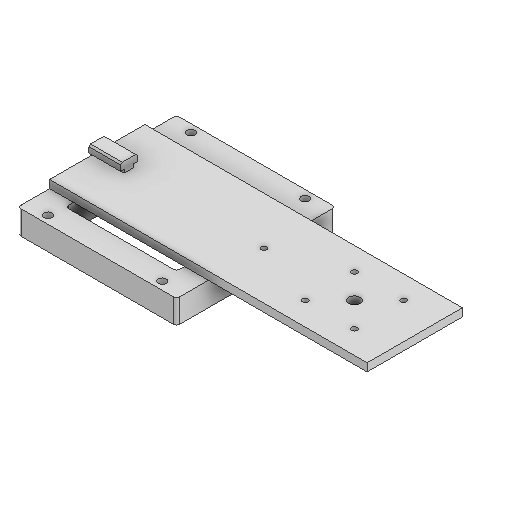
# Autodesk Inventor part: podstawka_prowadzaca
Saved by Autodesk Inventor 2025.1 (Build 291241000, 241)
## iProperties
Created: 2025-03-27
Part Number: podstawka_prowadzaca
Material: Ogólny
Document SubType Name: Modeling
Designer: Maciej
Density: 1 g/cm^3
Appearance: Domyślna
Author: Maciej
Autodesk Inventor part; units mm, degrees
ref_plane "YZ Plane" through (0, 0, 0) normal (1, 0, 0) x (0, 1, 0)
ref_plane "XZ Plane" through (0, 0, 0) normal (0, 1, 0) x (-1, 0, 0)
ref_plane "XY Plane" through (0, 0, 0) normal (0, 0, 1) x (1, 0, 0)
sketch "Szkic1" plane through (0, 0, 0) normal (0, 1, 0) x (-1, 0, 0)
  line L0 (0, 0) -> (100, 0)
  line L1 (100, 0) -> (100, -100)
  line L2 (100, -100) -> (0, -100)
  line L3 (0, -100) -> (0, 0)
  dimension "d0" = 100
  dimension "d1" = 100
  constraints: 8 end point, 2 parallel, 1 horizontal, 1 perpendicular
  measures "d0" distance of L0.end L1.end
  measures "d1" distance of L1.end L2.end
sketch "Szkic2" plane through (0, 0, 0) normal (0, 1, 0) x (-1, 0, 0)
  line L0 (15, -15) -> (85, -15)
  line L1 (85, -15) -> (85, -85)
  line L2 (85, -85) -> (15, -85)
  line L3 (15, -85) -> (15, -15)
  point P0 (0, 0)
  dimension "d2" = 70
  dimension "d3" = 70
  dimension "d4" = 15
  dimension "d5" = 15
  constraints: 8 end point, 2 parallel, 1 horizontal, 1 perpendicular
  measures "d2" distance of L1.end L2.end
  measures "d3" distance of L0.end L1.end
  measures "d4" horizontal distance of point (0, 0) L0.start
  measures "d5" horizontal distance of point (0, 0) L0.start
extrude "Wyciągnięcie proste1" add sketch "Szkic1" along normal blind 15
extrude "Wyciągnięcie proste2" cut sketch "Szkic2" along normal blind 15
fillet "Zaokrąglenie1" radius 2 8 edges at (-85, 7.5, -85) (-15, 7.5, -85) (-15, 7.5, -15) (-85, 7.5, -15) (-100, 7.5, 0) (-100, 7.5, -100) (0, 7.5, -100) (0, 7.5, 0)
sketch "Szkic3" plane through (0, 15, 0) normal (0, 1, 0) x (1, 0, 0)
  line L0 (0, 2) -> (0, 98) projected
  line L1 (-2, 100) -> (-98, 100) projected
  line L2 (-98, 0) -> (-2, 0) projected
  line L3 (-100, 98) -> (-100, 2) projected
  line L4 (-85, 17) -> (-85, 83) projected
  point P0 (0, 0)
  point P1 (-14, 95)
  point P2 (-14, 5)
  point P3 (-86, 95)
  point P4 (-86, 5)
  point P5 (-30, 100)
  point P6 (-100, 30)
  dimension "d12" = 5
  dimension "d13" = 5
  dimension "d14" = 5
  dimension "d18" = 5
  dimension "d32" = 14
  dimension "d33" = 14
  dimension "d34" = 14
  dimension "d35" = 14
  measures "d12" distance from line of L1 point (-14, 95)
  measures "d13" distance from line of L2 point (-14, 5)
  measures "d14" distance from line of L2 point (-86, 5)
  measures "d18" distance from line of L1 point (-86, 95)
  measures "d32" distance from line of L3 point (-86, 95)
  measures "d33" distance from line of L0 point (-14, 95)
  measures "d34" distance from line of L0 point (-14, 5)
  measures "d35" distance from line of L3 point (-86, 5)
hole "Otwór1" at (-14, 15, -95) at (-14, 15, -5) at (-86, 15, -95) at (-86, 15, -5) direction (0, -1, 0) diameter 5 depth 15 tip angle 118
sketch "Szkic4" plane through (0, 15, 0) normal (0, 1, 0) x (1, 0, 0)
  line L0 (-100, 98) -> (-100, 2) projected
  line L1 (-100, 20) -> (100, 20)
  line L2 (100, 20) -> (100, 80)
  line L3 (100, 80) -> (-100, 80)
  line L4 (-100, 80) -> (-100, 20)
  line L5 (-98, 0) -> (-2, 0) projected
  point P0 (0, 0)
  point P1 (-100, 80)
  point P2 (-100, 30)
  dimension "d26" = 60
  dimension "d29" = 20
  dimension "d30" = 200
  constraints: 8 end point, 2 parallel, 1 horizontal, 1 perpendicular, 1 point on line
  measures "d26" distance of L2.end L1.end
  measures "d29" distance between parallel lines of L5 L1
  measures "d30" distance of L2.end L3.end
extrude "Wyciągnięcie proste3" add sketch "Szkic4" along normal blind 5
sketch "Szkic5" plane through (-100, 0, -98) normal (-1, 0, 0) x (0, 0, 1)
  line L0 (48, 20) -> (44.975, 20)
  line L1 (18, 20) -> (78, 20) projected
  line L2 (44.975, 20) -> (44.975, 22)
  line L3 (44.975, 22) -> (42.75, 22)
  line L4 (42.75, 22) -> (42.75, 25.5)
  line L5 (48, 26.5) -> (43.75, 26.5)
  line L6 (43.75, 26.5) -> (42.75, 25.5)
  line L7 (48, 20) -> (51.025, 20)
  line L8 (51.025, 20) -> (51.025, 22)
  line L9 (51.025, 22) -> (53.25, 22)
  line L10 (53.25, 22) -> (53.25, 25.5)
  line L11 (48, 26.5) -> (52.25, 26.5)
  line L12 (52.25, 26.5) -> (53.25, 25.5)
  point P0 (98, 0)
  dimension "d36" = 3.025
  dimension "d37" = 2
  dimension "d38" = 2.225
  dimension "d39" = 3.5
  dimension "d40" = 6.5
  dimension "d41" = 4.25
  constraints: 24 end point, 2 perpendicular, 1 point on line, 1 vertical
  measures "d36" distance of L0.start L0.end
  measures "d37" distance of L0.end L2.end
  measures "d38" distance of L2.end L3.end
  measures "d39" distance of L3.end L4.end
  measures "d40" distance of L0.start L5.start
  measures "d41" distance of L5.start L5.end
extrude "Wyciągnięcie proste4" add sketch "Szkic5" against normal blind 20
sketch "Szkic6" plane through (0, 20, 0) normal (0, 1, 0) x (1, 0, 0)
  line L0 (0, 2) -> (0, 20) projected
  point P0 (0, 0)
  point P1 (5, 50)
  dimension "d51" = 5
  measures "d51" distance from line of L0 point (5, 50)
hole "Otwór2" at (5, 20, -50) direction (0, -1, 0) diameter 3.424 end through all
sketch "Szkic7" plane through (0, 20, 0) normal (0, 1, 0) x (1, 0, 0)
  circle A0 centre (5, 50) radius 1.712 projected
  point P0 (0, 0)
  point P1 (62, 50)
  dimension "d52" = 57
  measures "d52" distance of A0.centre point (62, 50)
hole "Otwór3" at (62, 20, -50) direction (0, -1, 0) diameter 7 end through all
sketch "Szkic8" plane through (0, 20, 0) normal (0, 1, 0) x (1, 0, 0)
  circle A0 centre (62, 50) radius 3.5 projected
  line L0 (46.5, 34.5) -> (77.5, 65.5) construction
  line L1 (77.5, 34.5) -> (46.5, 65.5) construction
  point P0 (0, 0)
  dimension "d60" = 31
  dimension "d61" = 31
  constraints: 4 coincident, 4 end point, 2 midpoint
  measures "d60" distance of L1.end L0.end
  measures "d61" distance of L0.end L1.start
hole "Otwór4" at (46.5, 20, -65.5) at (77.5, 20, -65.5) at (77.5, 20, -34.5) at (46.5, 20, -34.5) direction (0, -1, 0) diameter 3.4 end through all clearance for "Śruba ze łbem stożkowym ISO 2009/7046" size "M3" standard "ISO"
equation "\"d3\" = d2"
equation "\"d13\" = d12"
equation "\"d14\" = d12"
equation "\"d18\" = d12"
equation "\"d33\" = d32"
equation "\"d34\" = d32"
equation "\"d35\" = d32"
